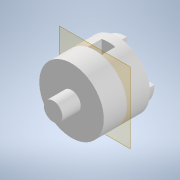
# Autodesk Inventor part: PotAttachmentB10L
Saved by Autodesk Inventor 2022 (Build 260153000, 153)
## iProperties
Created: 2021-10-23
Part Number: PotAttachmentB10L
Material: Generic
Document SubType Name: Modeling
Designer: teh18
Density: 1 g/cm^3
Appearance: Default
Author: teh18
Autodesk Inventor part; units mm, degrees
ref_plane "YZ Plane" through (0, 0, 0) normal (1, 0, 0) x (0, 1, 0)
ref_plane "XZ Plane" through (0, 0, 0) normal (0, 1, 0) x (-1, 0, 0)
ref_plane "XY Plane" through (0, 0, 0) normal (0, 0, 1) x (1, 0, 0)
sketch "Sketch1" plane through (0, 0, 0) normal (0, 0, 1) x (1, 0, 0)
  arc A0 (-0.1225, 6.9989) -> (-6, 3.6056) centre (0, 0) ccw projected
  circle A1 centre (0, 0) radius 7
  line L0 (0, -12) -> (0, -10) projected
  arc A2 (0, -10) -> (10, 0) centre (0, 0) ccw projected
  line L1 (10, 0) -> (12, 0) projected
  arc A3 (0, -12) -> (12, 0) centre (0, 0) ccw projected
  line L2 (0, 12) -> (0, 10) projected
  arc A4 (0, 10) -> (-10, 0) centre (0, 0) ccw projected
  line L3 (-10, 0) -> (-12, 0) projected
  arc A5 (0, 12) -> (-12, 0) centre (0, 0) ccw projected
  arc A6 (4.4269, -19.95) -> (6.1412, -19.4907) centre (5.1647, -19.275) ccw projected
  arc A7 (13.8088, -15.0638) -> (6.1412, -19.4907) centre (12, -20.7846) ccw projected
  arc A8 (13.8088, -15.0638) -> (15.0638, -13.8088) centre (14.1103, -14.1103) ccw projected
  arc A9 (19.4907, -6.1412) -> (15.0638, -13.8088) centre (20.7846, -12) ccw projected
  arc A10 (19.4907, -6.1412) -> (19.95, -4.4269) centre (19.275, -5.1647) ccw projected
  arc A11 (27.8571, 4.5959) -> (19.95, -4.4269) centre (24, 0) ccw projected
  arc A12 (27.8571, 4.5959) -> (29.4828, 5.5468) centre (28.5, 5.3619) ccw projected
  arc A13 (29.4828, 5.5468) -> (27.5804, 11.8035) centre (0, 0) ccw projected
  line L4 (27.5804, 11.8035) -> (33.0964, 14.1643) projected
  arc A14 (33.0964, 14.1643) -> (26.445, 24.4267) centre (0, 0) ccw projected
  line L5 (26.445, 24.4267) -> (22.0375, 20.3556) projected
  arc A15 (22.0375, 20.3556) -> (-20.3556, 22.0375) centre (0, 0) ccw projected
  line L6 (-20.3556, 22.0375) -> (-16.2845, 17.63) projected
  arc A16 (-16.2845, 17.63) -> (-5.9529, -23.25) centre (0, 0) ccw projected
  arc A17 (4.4269, -19.95) -> (-5.9529, -23.25) centre (0, -24) ccw projected
  arc A18 (-1, 6.9282) -> (-6.9282, 1) centre (0, 0) ccw projected
  line L7 (-1, 6.9282) -> (-1, 1) projected
  line L8 (-1, 1) -> (-6.9282, 1) projected
  line L9 (-6.9282, -1) -> (-1, -1) projected
  line L10 (-1, -1) -> (-1, -6.9282) projected
  arc A19 (-6.9282, -1) -> (-1, -6.9282) centre (0, 0) ccw projected
  line L11 (1, -6.9282) -> (1, -1) projected
  line L12 (1, -1) -> (6.9282, -1) projected
  arc A20 (1, -6.9282) -> (6.9282, -1) centre (0, 0) ccw projected
  line L13 (6.9282, 1) -> (1, 1) projected
  line L14 (1, 1) -> (1, 6.9282) projected
  arc A21 (6.9282, 1) -> (1, 6.9282) centre (0, 0) ccw projected
  circle A22 centre (0, 0) radius 14
  point P0 (0, 0)
  point P1 (-6, 3.6056)
  point P2 (-0.1225, 6.9989)
  dimension "d2" = 28
  constraints: 1 centre point, 1 coincident, 2 other
  measures "d2" diameter of A22
extrude "Extrusion1" add sketch "Sketch1" along normal blind 20 contours L0 A2 L1 A3 | L2 A4 L3 A5 | A22
sketch "Sketch2" plane through (0, 0, 0) normal (0, 0, -1) x (-1, 0, 0)
  line L0 (0, -12) -> (0, -10) projected
  arc A0 (-10, 0) -> (0, -10) centre (0, 0) ccw projected
  line L1 (-10, 0) -> (-12, 0) projected
  arc A1 (-12, 0) -> (0, -12) centre (0, 0) ccw projected
  line L2 (0, 12) -> (0, 10) projected
  arc A2 (10, 0) -> (0, 10) centre (0, 0) ccw projected
  line L3 (10, 0) -> (12, 0) projected
  arc A3 (12, 0) -> (0, 12) centre (0, 0) ccw projected
  arc A4 (-6.1412, -19.4907) -> (-4.4269, -19.95) centre (-5.1647, -19.275) ccw projected
  arc A5 (-6.1412, -19.4907) -> (-13.8088, -15.0638) centre (-12, -20.7846) ccw projected
  arc A6 (-15.0638, -13.8088) -> (-13.8088, -15.0638) centre (-14.1103, -14.1103) ccw projected
  arc A7 (-15.0638, -13.8088) -> (-19.4907, -6.1412) centre (-20.7846, -12) ccw projected
  arc A8 (-19.95, -4.4269) -> (-19.4907, -6.1412) centre (-19.275, -5.1647) ccw projected
  arc A9 (-19.95, -4.4269) -> (-27.8571, 4.5959) centre (-24, 0) ccw projected
  arc A10 (-29.4828, 5.5468) -> (-27.8571, 4.5959) centre (-28.5, 5.3619) ccw projected
  arc A11 (-27.5804, 11.8035) -> (-29.4828, 5.5468) centre (0, 0) ccw projected
  line L4 (-27.5804, 11.8035) -> (-33.0964, 14.1643) projected
  arc A12 (-26.445, 24.4267) -> (-33.0964, 14.1643) centre (0, 0) ccw projected
  line L5 (-26.445, 24.4267) -> (-22.0375, 20.3556) projected
  arc A13 (20.3556, 22.0375) -> (-22.0375, 20.3556) centre (0, 0) ccw projected
  line L6 (20.3556, 22.0375) -> (16.2845, 17.63) projected
  arc A14 (5.9529, -23.25) -> (16.2845, 17.63) centre (0, 0) ccw projected
  arc A15 (5.9529, -23.25) -> (-4.4269, -19.95) centre (0, -24) ccw projected
  arc A16 (6.9282, 1) -> (1, 6.9282) centre (0, 0) ccw projected
  line L7 (1, 6.9282) -> (1, 1) projected
  line L8 (1, 1) -> (6.9282, 1) projected
  line L9 (6.9282, -1) -> (1, -1) projected
  line L10 (1, -1) -> (1, -6.9282) projected
  arc A17 (1, -6.9282) -> (6.9282, -1) centre (0, 0) ccw projected
  line L11 (-1, -6.9282) -> (-1, -1) projected
  line L12 (-1, -1) -> (-6.9282, -1) projected
  arc A18 (-6.9282, -1) -> (-1, -6.9282) centre (0, 0) ccw projected
  line L13 (-6.9282, 1) -> (-1, 1) projected
  line L14 (-1, 1) -> (-1, 6.9282) projected
  arc A19 (-1, 6.9282) -> (-6.9282, 1) centre (0, 0) ccw projected
  point P0 (0, 0)
extrude "Extrusion2" add sketch "Sketch2" along normal blind 4 contours A1 L1 A0 L0 | A3 L3 A2 L2
ref_plane "Work Plane1" through (0, 0, 10) normal (0, 0, 1) x (1, 0, 0)
sketch "Sketch4" plane through (0, 0, 10) normal (0, 0, 1) x (1, 0, 0)
  circle A0 centre (0, 0) radius 3
  circle A1 centre (0, 0) radius 7 projected
  dimension "d10" = 6
  constraints: 1 centre point, 1 coincident
  measures "d10" diameter of A0
extrude "Extrusion4" add sketch "Sketch4" along normal up to surface (10 mm away) contours A0 | A1
sketch "Sketch6" plane through (0, 0, 20) normal (0, 0, 1) x (1, 0, 0)
  circle A0 centre (0, 0) radius 4
  dimension "d25" = 8
  constraints: 1 centre point, 1 coincident
  measures "d25" diameter of A0
extrude "Extrusion6" add sketch "Sketch6" along normal blind 8
sketch "Sketch5" plane through (0, 0, 10) normal (0, 0, 1) x (1, 0, 0)
  line L0 (-3, 24.9703) -> (3, 24.9703)
  line L1 (3, 24.9703) -> (3, 3)
  line L2 (3, 3) -> (-3, 3)
  line L3 (-3, 3) -> (-3, 24.9703)
  line L4 (-3, 24.9703) -> (3, 3) construction
  line L5 (3, 24.9703) -> (-3, 3) construction
  arc A0 (3, 0) -> (3, 0) centre (0, 0) ccw projected
  circle A1 centre (0, 0) radius 14 projected
  point P0 (0, 13.9851)
  point P1 (0, 24.9703)
  dimension "d14" = 6
  constraints: 12 end point, 3 midpoint, 2 parallel, 1 horizontal, 1 perpendicular
  measures "d14" distance of L1.end L2.end
extrude "Extrusion5" cut sketch "Sketch5" against normal blind 6 contours L0 L1 A1 L3 | A1 L1 L2 L3 picked at (2, 6.5583)
spur gear teeth "Spur Gear2" teeth 15 pitch diameter 15 tip diameter 17 root diameter 12.5 face width 8 trims to tip circle yes start plane through (0, 0, 20) normal (0, 0, 1) x (1, 0, 0)
body "Solid1"
